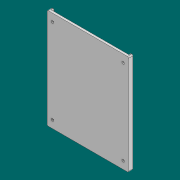
# Autodesk Inventor part: bottom_140mm_3
Saved by Autodesk Inventor 2022 (Build 260153000, 153)
## iProperties
Created: 2022-10-11
Part Number: bottom_140mm_3
Material: 一般
Document SubType Name: Modeling
Designer: numai
Density: 1 g/cm^3
Appearance: 既定
Author: numai
Autodesk Inventor part; units mm, degrees
ref_plane "YZ Plane" through (0, 0, 0) normal (1, 0, 0) x (0, 1, 0)
ref_plane "XZ Plane" through (0, 0, 0) normal (0, 1, 0) x (-1, 0, 0)
ref_plane "XY Plane" through (0, 0, 0) normal (0, 0, 1) x (1, 0, 0)
sketch "スケッチ1" plane through (0, 0, 0) normal (0, 0, 1) x (1, 0, 0)
  line L0 (-75, 92) -> (75, 92)
  line L1 (75, 92) -> (75, -92)
  line L2 (75, -92) -> (-75, -92)
  line L3 (-75, -92) -> (-75, 92)
  line L4 (65, 92) -> (65, -92) construction
  line L5 (-65, 92) -> (-65, -92) construction
  line L6 (-65, 0) -> (65, 0) construction
  circle A0 centre (-65, 78) radius 2.25
  circle A1 centre (65, 78) radius 2.25
  circle A2 centre (-65, -78) radius 2.25
  circle A3 centre (65, -78) radius 2.25
  point P0 (0, 0)
  point P1 (0, 92)
  point P2 (-75, 0)
  point P3 (0, 0)
  dimension "d0" = 184
  dimension "d1" = 150
  dimension "d2" = 130
  dimension "d3" = 78
  dimension "d4" = 78
  dimension "d5" = 4.5
  constraints: 14 end point, 8 point on line, 5 midpoint, 4 centre point, 3 equal radius, 3 horizontal alignment, 3 perpendicular, 2 parallel, 1 coincident, 1 horizontal, 1 vertical alignment
  measures "d0" distance of L2.end L0.start
  measures "d1" distance of L0.start L0.end
  measures "d2" distance between parallel lines of L4 L5
  measures "d3" vertical distance of point (0, 0) A0.centre
  measures "d4" distance from line of A2.centre L6
  measures "d5" diameter of A0
extrude "押し出し1" add sketch "スケッチ1" along normal blind 4
sketch "スケッチ3" plane through (0, 0, 0) normal (0, 0, 1) x (1, 0, 0)
  line L0 (-75, -92) -> (75, -92) construction
  line L1 (-75, 92) -> (-75, -92) construction
  line L2 (75, 92) -> (-75, 92) construction
  line L3 (75, -92) -> (75, 92) construction
  circle A0 centre (65, -78) radius 2.25 construction
  circle A1 centre (-65, -78) radius 2.25 construction
  circle A2 centre (65, 78) radius 2.25 construction
  circle A3 centre (-65, 78) radius 2.25 construction
  line L4 (75, 92) -> (-75, 92) projected
  line L5 (-75, -92) -> (75, -92) projected
  line L6 (-75, 92) -> (-70, 92)
  line L7 (-70, 92) -> (-70, -92)
  line L8 (-70, -92) -> (-75, -92)
  line L9 (-75, -92) -> (-75, 92)
  line L10 (75, -92) -> (75, 92) projected
  line L11 (75, 92) -> (70, 92)
  line L12 (70, 92) -> (70, -92)
  line L13 (70, -92) -> (75, -92)
  line L14 (75, -92) -> (75, 92)
  point P0 (0, 0)
  point P1 (70, 92)
  point P2 (70, -92)
  dimension "d8" = 5
  constraints: 16 end point, 4 parallel, 2 horizontal, 2 perpendicular, 2 point on line, 1 collinear
  measures "d8" distance between parallel lines of L1 L7
extrude "押し出し2" add sketch "スケッチ3" against normal blind 4 contours L10 L5 L12 L4 | L7 L5 L9 L4
sketch "スケッチ4" plane through (0, 0, 0) normal (0, 0, -1) x (-1, 0, 0)
  circle A0 centre (65, 78) radius 2.25 construction
  circle A1 centre (-65, 78) radius 2.25 construction
  circle A2 centre (-65, -78) radius 2.25 construction
  circle A3 centre (65, -78) radius 2.25 construction
  circle A4 centre (65, 78) radius 2.25 projected
  circle A5 centre (65, 78) radius 4.25
  circle A6 centre (65, -78) radius 2.25 projected
  circle A7 centre (65, -78) radius 4.25
  circle A8 centre (-65, 78) radius 2.25 projected
  circle A9 centre (-65, 78) radius 4.25
  circle A10 centre (-65, -78) radius 2.25 projected
  circle A11 centre (-65, -78) radius 4.25
  point P0 (0, 0)
  point P1 (63.9692, 92)
  point P2 (66.0308, 92)
  point P3 (-66.0308, 92)
  point P4 (-63.9692, 92)
  point P5 (-63.9692, -92)
  point P6 (-66.0308, -92)
  point P7 (66.0308, -92)
  point P8 (63.9692, -92)
  dimension "d12" = 8.5
  constraints: 4 centre point, 4 coincident, 3 equal radius, 8 other
  measures "d12" diameter of A5
extrude "押し出し3" cut sketch "スケッチ4" against normal blind 1.5 contours A4 | A5 | A6 | A7 | A8 | A9 | A10 | A11
fillet "フィレット1" radius 2 8 edges at (-70, 92, -2) (-75, 92, 0) (70, 92, -2) (75, 92, 0) (75, -92, 0) (70, -92, -2) (-70, -92, -2) (-75, -92, 0)
equation "\"d4\" = d3"
